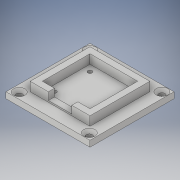
# Autodesk Inventor part: PigeonIMUMount
Saved by Autodesk Inventor 2019 (Build 230136000, 136)
## iProperties
Created: 2018-01-17
Part Number: PigeonIMUMount
Material: Generic
Document SubType Name: Modeling
Designer: james
Density: 1 g/cm^3
Appearance: Default
Mass: 31.373 g
Surface Area: 143.674 cm^2
Volume: 31.373 cm^3
Author: james
Autodesk Inventor part; units mm, degrees
ref_plane "YZ Plane" through (0, 0, 0) normal (1, 0, 0) x (0, 1, 0)
ref_plane "XZ Plane" through (0, 0, 0) normal (0, 1, 0) x (-1, 0, 0)
ref_plane "XY Plane" through (0, 0, 0) normal (0, 0, 1) x (1, 0, 0)
sketch "Sketch1" plane through (0, 0, 0) normal (0, 1, 0) x (-1, 0, 0)
  line L0 (17.7305, 21.844) -> (-22.2695, 21.844)
  line L1 (-22.2695, 21.844) -> (-22.2695, -18.156)
  line L2 (-22.2695, -18.156) -> (17.7305, -18.156)
  line L3 (17.7305, -18.156) -> (17.7305, 21.844)
  line L4 (22.8105, 26.924) -> (-27.3495, 26.924)
  line L5 (-27.3495, 26.924) -> (-27.3495, -23.236)
  line L6 (-27.3495, -23.236) -> (22.8105, -23.236)
  line L7 (22.8105, -23.236) -> (22.8105, 26.924)
  point P0 (0, 0)
  dimension "d0" = 40
  dimension "d1" = 40
  dimension "d2" = 5.08
  dimension "d3" = 5.08
  dimension "d4" = 5.08
  dimension "d5" = 5.08
  constraints: 16 end point, 4 parallel, 2 horizontal, 2 perpendicular
  measures "d0" distance of L0.start L0.end
  measures "d1" distance of L2.end L0.start
  measures "d2" distance between parallel lines of L2 L6
  measures "d3" distance between parallel lines of L7 L3
  measures "d4" distance between parallel lines of L4 L0
  measures "d5" distance between parallel lines of L1 L5
extrude "Extrusion1" add sketch "Sketch1" along normal blind 7.62
sketch "Sketch2" plane through (0, 0, 0) normal (0, -1, 0) x (1, 0, 0)
  line L0 (37.5095, 37.084) -> (-32.9705, 37.084)
  line L1 (-32.9705, 37.084) -> (-32.9705, -33.396)
  line L2 (-32.9705, -33.396) -> (37.5095, -33.396)
  line L3 (37.5095, -33.396) -> (37.5095, 37.084)
  line L4 (-22.8105, 26.924) -> (27.3495, 26.924) projected
  line L5 (27.3495, 26.924) -> (27.3495, -23.236) projected
  line L6 (-22.8105, -23.236) -> (-22.8105, 26.924) projected
  line L7 (27.3495, -23.236) -> (-22.8105, -23.236) projected
  point P0 (0, 0)
  dimension "d8" = 10.16
  dimension "d9" = 10.16
  dimension "d10" = 10.16
  dimension "d11" = 10.16
  constraints: 8 end point, 2 parallel, 1 horizontal, 1 perpendicular
  measures "d8" distance between parallel lines of L0 L4
  measures "d9" distance between parallel lines of L5 L3
  measures "d10" distance between parallel lines of L6 L1
  measures "d11" distance between parallel lines of L7 L2
extrude "Extrusion2" add sketch "Sketch2" along normal blind 5.08 contours L3 L2 L1 L0 | L4 L5 L7 L6
sketch "Sketch3" plane through (0, 0, 0) normal (0, 1, 0) x (1, 0, 0)
  line L0 (-32.9705, 33.396) -> (37.5095, 33.396) projected
  line L1 (-32.9705, -37.084) -> (-32.9705, 33.396) projected
  line L2 (37.5095, 33.396) -> (37.5095, -37.084) projected
  line L3 (37.5095, -37.084) -> (-32.9705, -37.084) projected
  point P0 (0, 0)
  point P1 (-27.8905, 28.316)
  point P2 (32.4295, 28.3337)
  point P3 (31.8578, -32.004)
  point P4 (-27.206, -31.7168)
  dimension "d14" = 5.08
  dimension "d15" = 5.08
  dimension "d16" = 5.08
  dimension "d17" = 5.08
  measures "d14" distance from line of L0 point (-27.89, 28.316)
  measures "d15" distance from line of L1 point (-27.89, 28.316)
  measures "d16" distance from line of L2 point (32.43, 28.334)
  measures "d17" distance from line of L3 point (31.858, -32.004)
hole "Hole1" at (-27.8905, 0, -28.316) at (32.4295, 0, -28.3337) at (31.8578, 0, 32.004) at (-27.206, 0, 31.7168) direction (0, -1, 0) diameter 5.08 depth 25.4 tip angle 118 countersink diameter 9.525 countersink angle 82
sketch "Sketch4" plane through (0, 0, 0) normal (0, 1, 0) x (1, 0, 0)
  line L0 (-17.7305, 18.156) -> (22.2695, 18.156) projected
  line L1 (22.2695, -21.844) -> (-17.7305, -21.844) projected
  line L2 (22.2695, -21.844) -> (22.2695, 18.156) projected
  line L3 (-17.7305, 18.156) -> (-17.7305, -21.844) projected
  point P0 (0, 0)
  point P1 (-12.2305, 12.656)
  point P2 (16.7695, 12.656)
  point P3 (16.7695, -16.344)
  point P4 (-12.7285, -16.7964)
  dimension "d25" = 29
  dimension "d26" = 29
  dimension "d27" = 5.5
  dimension "d28" = 5.5
  dimension "d29" = 5.5
  dimension "d30" = 5.5
  measures "d25" distance of point (-12.23, 12.656) point (16.77, 12.656)
  measures "d26" distance of point (16.77, -16.344) point (16.77, 12.656)
  measures "d27" distance from line of L0 point (16.77, 12.656)
  measures "d28" distance from line of L1 point (16.77, -16.344)
  measures "d29" distance from line of L2 point (16.77, -16.344)
  measures "d30" distance from line of L3 point (-12.23, 12.656)
hole "Hole2" at (-12.2305, 0, -12.656) at (16.7695, 0, -12.656) at (16.7695, 0, 16.344) at (-12.7285, 0, 16.7964) direction (0, -1, 0) diameter 3.5 depth 25.4 tip angle 118
sketch "Sketch5" plane through (0, 7.62, 0) normal (0, 1, 0) x (1, 0, 0)
  line L0 (-7.5705, -40.5496) -> (12.1095, -40.5496)
  line L1 (12.1095, -40.5496) -> (12.1095, -14.6017)
  line L2 (12.1095, -14.6017) -> (-7.5705, -14.6017)
  line L3 (-7.5705, -14.6017) -> (-7.5705, -40.5496)
  line L4 (-22.8105, 23.236) -> (-22.8105, -26.924) projected
  line L5 (27.3495, -26.924) -> (27.3495, 23.236) projected
  point P0 (0, 0)
  dimension "d38" = 15.24
  dimension "d39" = 15.24
  constraints: 8 end point, 2 parallel, 1 horizontal, 1 perpendicular
  measures "d38" distance between parallel lines of L3 L4
  measures "d39" distance between parallel lines of L5 L1
extrude "Extrusion3" cut sketch "Sketch5" against normal blind 6.35
body "Solid1"
